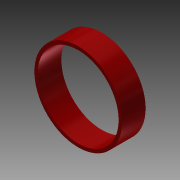
# Autodesk Inventor part: Tread
Saved by Autodesk Inventor 2013 (Build 170138000, 138)
## iProperties
Created: 2013-04-01
Part Number: Tread
Material: Generic
Document SubType Name: Modeling
Designer: mvarma
Density: 1 g/cm^3
Author: mvarma
Autodesk Inventor part; units mm, degrees
ref_plane "YZ Plane" through (0, 0, 0) normal (1, 0, 0) x (0, 1, 0)
ref_plane "XZ Plane" through (0, 0, 0) normal (0, 1, 0) x (-1, 0, 0)
ref_plane "XY Plane" through (0, 0, 0) normal (0, 0, 1) x (1, 0, 0)
sketch "Sketch1" plane through (0, 0, 0) normal (0, 0, 1) x (1, 0, 0)
  circle A0 centre (0, 0) radius 38.1
  circle A1 centre (0, 0) radius 41.275
  dimension "d0" = 76.2
  dimension "d2" = 82.55
  constraints: 2 centre point, 2 coincident
  measures "d0" diameter of A0
  measures "d2" diameter of A1
extrude "Extrusion1" add sketch "Sketch1" along normal blind 22.225
body "Solid1"
